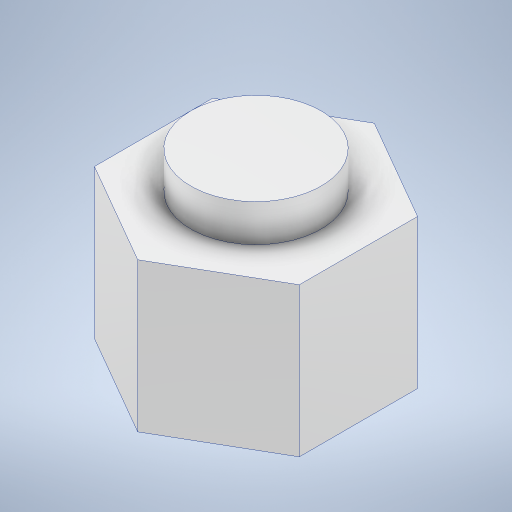
# Autodesk Inventor part: EccentricNut 5mmID 11mmHex
Saved by Autodesk Inventor 2023 (Build 270158000, 158)
## iProperties
Created: 2023-04-10
Part Number: EccentricNut 5mmID 11mmHex
Material: Aluminum 6061
Document SubType Name: Modeling
Designer: ethan
Density: 2.7 g/cm^3
Appearance: Aluminum - Flat
Author: ethan
Autodesk Inventor part; units mm, degrees
ref_plane "YZ Plane" through (0, 0, 0) normal (1, 0, 0) x (0, 1, 0)
ref_plane "XZ Plane" through (0, 0, 0) normal (0, 1, 0) x (-1, 0, 0)
ref_plane "XY Plane" through (0, 0, 0) normal (0, 0, 1) x (1, 0, 0)
sketch "Sketch1" plane through (0, 0, 0) normal (0, 1, 0) x (-1, 0, 0)
  line L0 (5.5, -3.1754) -> (0, -6.3509)
  line L1 (0, -6.3509) -> (-5.5, -3.1754)
  line L2 (-5.5, -3.1754) -> (-5.5, 3.1754)
  line L3 (-5.5, 3.1754) -> (0, 6.3509)
  line L4 (0, 6.3509) -> (5.5, 3.1754)
  line L5 (5.5, 3.1754) -> (5.5, -3.1754)
  circle A0 centre (0, 0) radius 3.5
  dimension "d0" = 7
  dimension "d1" = 11
  constraints: 12 end point, 2 coincident, 1 centre point, 1 vertical, 13 other
  measures "d0" diameter of A0
  measures "d1" distance between parallel lines of L2 L5
extrude "Extrusion1" add sketch "Sketch1" against normal blind 8 contours L0 L1 L2 L3 L4 L5 | A0
extrude "Extrusion2" add sketch "Sketch1" along normal blind 2 contours A0
body "Solid1"
